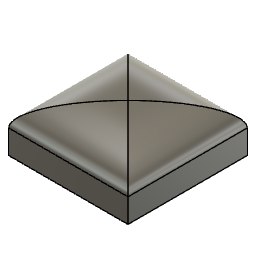
Task3 v1 (Autodesk Fusion 360 design; units mm, degrees)
Autodesk Fusion 360 part; units mm, degrees
note: some values were not read from the file. Set by a fixed rule: which sketch regions a step uses.
sketch "Sketch1" plane through (0, 0, 0) normal (0, 1, 0) x (1, 0, 0)
  line L0 (50, -50) -> (-50, -50)
  line L1 (-50, -50) -> (-50, 50)
  line L2 (-50, 50) -> (50, 50)
  line L3 (50, 50) -> (50, -50)
  line L4 (50, -50) -> (-50, 50) construction
  line L5 (-50, -50) -> (50, 50) construction
  dimension "d1" = 100
  dimension "d2" = 100
  constraint horizontal L0
  constraint perpendicular L0 L1
  constraint parallel L0 L2
  constraint parallel L1 L3
  constraint coincident L4 origin
  constraint coincident L5 origin
  measures "d1" distance of L1.end L2.end
  measures "d2" distance of L0.end L1.end
extrude "Extrude1" add sketch "Sketch1" along normal blind 20 makes body 1
sketch "Sketch2" plane through (0, 0, -50) normal (0, 0, -1) x (-1, 0, 0)
  line L0 (-50, 0) -> (50, 0)
  line L1 (50, 0) -> (50, 20)
  line L2 (50, 20) -> (-50, 20)
  line L3 (-50, 20) -> (-50, 0)
  ellipse E0 centre (0, 20) end of major axis (50, 20) minor radius 20
  line L4 (-50, 20) -> (50, 20)
  line L5 (0, 0) -> (0, 40)
  dimension "d5" = 40
  constraint midpoint L2 E0.centre
  constraint coincident L2.end E0
  constraint coincident L1.end E0
  constraint coincident E0 L5.end
extrude "Extrude2" add sketch "Sketch2" against normal blind 100 separate body contours L2 E0 L4 L5 | L2 E0 L4 L5 picked at (-29.3498, 24.3251) picked at (27.8267, 24.9515) makes body 2
sketch "Sketch3" plane through (-50, 0, 0) normal (-1, 0, 0) x (0, 0, 1)
  line L0 (-50, 0) -> (50, 0)
  line L1 (50, 0) -> (50, 20)
  line L2 (50, 20) -> (-50, 20)
  line L3 (-50, 20) -> (-50, 0)
  ellipse E0 centre (0, 20) end of major axis (50, 20) minor radius 20
  line L4 (-50, 20) -> (50, 20)
  line L5 (0, 0) -> (0, 40)
  dimension "d8" = 40
  constraint midpoint L2 E0.centre
  constraint coincident L2.end E0
  constraint coincident L5.start E0
extrude "Extrude3" add sketch "Sketch3" against normal blind 100 separate body contours L2 E0 L4 L5 | L2 E0 L4 L5 picked at (-29.3498, 24.3251) picked at (27.8267, 24.9515) makes body 3
sketch "Sketch4" plane through (0, 0, 0) normal (0, -1, 0) x (1, 0, 0)
  line L0 (-50, -50) -> (50, -50)
  line L1 (50, -50) -> (50, 50)
  line L2 (50, 50) -> (-50, 50)
  line L3 (-50, 50) -> (-50, -50)
  line L4 (50, 50) -> (-50, -50)
  line L5 (-50, 50) -> (50, -50)
  constraint coincident L1.end L2.start
  constraint coincident L0.start L3.end
  constraint coincident L2.end L3.start
  constraint coincident L0.end L1.start
extrude "Extrude4" cut sketch "Sketch4" along normal blind -20 and the other way blind 40 contours L0 L4 L5 | L2 L4 L5 bodies 2
extrude "Extrude5" cut sketch "Sketch4" along normal blind -20 and the other way blind 40 contours L3 L4 L5 | L1 L4 L5 bodies 3
combine "Combine1" operation add target body 1 tool bodies 2 3
